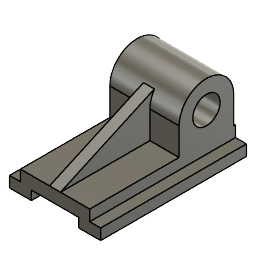
Untitled11 (Autodesk Fusion 360 design; units mm, degrees)
part number: 2026-08-20-00-34-06-763
Autodesk Fusion 360 part; units mm, degrees
sketch "Sketch1" plane through (0, 0, 0) normal (0, 1, 0) x (1, 0, 0)
  line L0 (50, 80) -> (-50, 80)
  line L1 (-50, 80) -> (-50, -80)
  line L2 (-50, -80) -> (50, -80)
  line L3 (50, -80) -> (50, 80)
  line L4 (50, 80) -> (-50, -80) construction
  line L5 (-50, 80) -> (50, -80) construction
  line L6 (38, -80) -> (38, 80)
  line L7 (26, -80) -> (26, 80)
  line L8 (-38, 80) -> (-38, -80)
  line L9 (-26, 80) -> (-26, -80)
  dimension "d1" = 100
  dimension "d2" = 160
  dimension "d3" = 12
  dimension "d4" = 12
  dimension "d5" = 12
  dimension "d6" = 12
  constraint horizontal L0
  constraint perpendicular L0 L1
  constraint parallel L0 L2
  constraint parallel L1 L3
  constraint coincident L4 origin
  constraint coincident L5 origin
  constraint coincident L2 L6.start
  constraint coincident L0 L6.end
  constraint perpendicular L0 L6
  constraint coincident L2 L7.start
  constraint coincident L0 L7.end
  constraint perpendicular L0 L7
  constraint coincident L0 L8.start
  constraint coincident L2 L8.end
  constraint perpendicular L2 L8
  constraint coincident L0 L9.start
  constraint perpendicular L0 L9
  constraint equal L8 L9
  measures "d1" distance of L1.end L2.end
  measures "d2" distance of L0.end L1.end
  measures "d3" distance of L2.end L6.start
  measures "d4" distance of L6.start L7.start
  measures "d5" distance of L8.end L9.end
  measures "d6" distance of L1.end L8.end
extrude "Extrude1" add sketch "Sketch1" along normal blind 24 contours L0 L2 L6 L7 | L0 L2 L7 L9 | L0 L2 L8 L9 makes body 1
extrude "Extrude2" add sketch "Sketch1" along normal blind 12 separate body contours L0 L2 L3 L6 | L0 L1 L2 L8 makes body 2 at (-38, 4, -26.6667) makes body 3 at (42, 0, -26.6667)
sketch "Sketch2" plane through (0, 0, 80) normal (0, 0, 1) x (1, 0, 0)
  line L0 (-38, 0) -> (38, 0)
  line L1 (38, 0) -> (38, 24)
  line L2 (38, 24) -> (-38, 24)
  line L3 (-38, 24) -> (-38, 0)
  line L4 (-26, 0) -> (26, 0)
  line L5 (26, 0) -> (26, 10)
  line L6 (26, 10) -> (-26, 10)
  line L7 (-26, 10) -> (-26, 0)
  dimension "d11" = 52
  dimension "d12" = 10
  constraint horizontal L4
  constraint vertical L5
  constraint horizontal L6
  constraint vertical L7
  constraint coincident L0 L4.start
  measures "d11" distance of L4.start L4.end
  measures "d12" distance of L4.start L6.end
extrude "Extrude3" cut sketch "Sketch2" against normal blind 160 contours L0 L4 L5 L6 L7 bodies 1
sketch "Sketch3" plane through (38, 0, 0) normal (1, 0, 0) x (0, 0, -1)
  line L0 (-80, 0) -> (80, 0)
  line L1 (80, 0) -> (80, 24)
  line L2 (80, 24) -> (-80, 24)
  line L3 (-80, 24) -> (-80, 0)
  line L4 (78.0118, 24) -> (18.0118, 24)
  line L5 (18.0118, 24) -> (18.0118, 54)
  line L6 (78.0118, 54) -> (78.0118, 24)
  circle A0 centre (48.0118, 54) radius 15
  arc A1 (78.0118, 54) -> (18.0118, 54) centre (48.0118, 54) ccw
  dimension "d15" = 60
  dimension "d17" = 60
  dimension "d18" = 30
  constraint horizontal L4
  constraint vertical L5
  constraint vertical L6
  constraint coincident L2 L4.start
  constraint concentric A0 A1
  measures "d15" distance of L4.start L4.end
  measures "d17" diameter of A1
  measures "d18" diameter of A0
extrude "Extrude4" add sketch "Sketch3" against normal blind 76 contours L2 L4 L5 L6 A1 bodies 1
sketch "Sketch4" plane through (0, 24, 0) normal (0, 1, 0) x (-1, 0, 0)
  line L0 (-38, -18.0118) -> (38, -18.0118)
  line L1 (38, -18.0118) -> (38, 80)
  line L2 (38, 80) -> (-38, 80)
  line L3 (-38, 80) -> (-38, -18.0118)
  line L4 (-6, 80) -> (-6, -20)
  line L5 (-6, -20) -> (6, -20)
  line L6 (6, -20) -> (6, 80)
  line L7 (6, 80) -> (-6, 80)
  dimension "d21" = 100
  dimension "d22" = 12
  dimension "d23" = 100
  constraint coincident L2 L4.start
  constraint perpendicular L4 L5
  constraint vertical L6
  constraint perpendicular L4 L7
  measures "d21" distance of L4.start L4.end
  measures "d22" distance of L4.end L5.end
  measures "d23" distance of L5.end L6.end
extrude "Extrude5" add sketch "Sketch4" along normal blind 75 contours L0 L2 L4 L6 L7 bodies 1
sketch "Sketch5" plane through (6, 0, 0) normal (1, 0, 0) x (0, 0, -1)
  line L0 (-80, 24) -> (18.0118, 24)
  line L1 (18.0118, 24) -> (18.0118, 54)
  line L2 (18.0118, 54) -> (18.0118, 99)
  line L3 (18.0118, 99) -> (-80, 99)
  line L4 (-80, 99) -> (-80, 24)
  line L5 (-80, 25) -> (18.0118, 76.5)
  line L6 (18.0118, 76.5) -> (18.0118, 25)
  constraint coincident L4 L5.start
  constraint midpoint L2 L5.end
  constraint coincident L1 L6.end
extrude "Extrude6" cut sketch "Sketch5" against normal blind 12 contours L2 L3 L4 L5 bodies 1
move_face "OffsetFaces1" offset 5 1 faces at (-2, 69, -18.0118) on bodies 1
sketch "Sketch6" plane through (6, 0, 0) normal (1, 0, 0) x (0, 0, -1)
  arc A0 (23.0118, 70.5831) -> (18.0118, 54) centre (48.0118, 54) ccw
  line L0 (23.0118, 70.5831) -> (23.0118, 79.1272)
  line L1 (23.0118, 79.1272) -> (-80, 25)
  line L2 (-80, 25) -> (-80, 24)
  line L3 (-80, 24) -> (18.0118, 24)
  line L4 (18.0118, 24) -> (18.0118, 54)
  line L5 (-80, 24) -> (23.0118, 70.5831)
  constraint coincident L2.end L3.start
  constraint coincident A0.start L0.start
extrude "Extrude7" cut sketch "Sketch6" against normal blind 12 contours L0 L1 L2 L5 bodies 1
combine "Combine1" operation add target body 3 tool bodies 2 1
